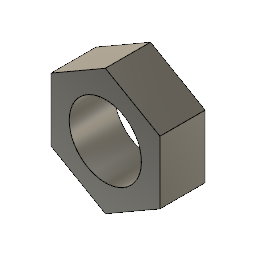
assembly v43 (Autodesk Fusion 360 archive; units mm, degrees)
design "nut"
Autodesk Fusion 360 part; units mm, degrees
sketch "Sketch1" plane through (0, 0, 0) normal (0, 1, 0) x (1, 0, 0)
  circle A0 centre (0, 0) radius 1.75
  line L0 (2.65, 1.53) -> (0, 3.06)
  line L1 (0, 3.06) -> (-2.65, 1.53)
  line L2 (-2.65, 1.53) -> (-2.65, -1.53)
  line L3 (-2.65, -1.53) -> (0, -3.06)
  line L4 (0, -3.06) -> (2.65, -1.53)
  line L5 (2.65, -1.53) -> (2.65, 1.53)
  dimension "d1" = 3.5
  dimension "d2" = 5.3
  constraint coincident A0.centre origin
  measures "d1" diameter of A0
  measures "d2" distance of L2 L5
extrude "Extrude1" add sketch "Sketch1" along normal blind 2.2

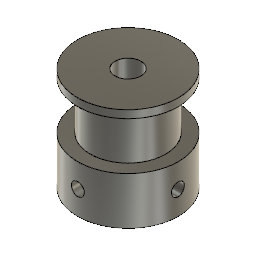
design "motor pulley"
Autodesk Fusion 360 part; units mm, degrees
sketch "Sketch1" plane through (0, 0, 0) normal (0, 0, 1) x (1, 0, 0)
  circle A0 centre (0, 0) radius 7.85
  circle A1 centre (0, 0) radius 2
  dimension "d1" = 15.7
  dimension "d4" = 4
  constraint coincident A0.centre A1.centre
  constraint concentric A0 A1
  measures "d1" diameter of A0
  measures "d4" diameter of A1
extrude "Extrude1" add sketch "Sketch1" along normal blind 16 makes body 1
copy_body "Body->Comp1" bodies 1 removing the originals makes body 2 in component "Component"
sketch "Sketch3" plane through (0, 0, 16) normal (0, 0, 1) x (-1, 0, 0)
  circle A0 centre (0, 0) radius 2
  circle A1 centre (0, 0) radius 7.85
  circle A2 centre (0, 0) radius 5.85
  dimension "d6" = 2
  constraint coincident A0.centre A1.centre
  measures "d6" distance of A1 A2
extrude "Extrude1'" cut sketch "Sketch3" against normal blind 7.4 from surface at -1.2 contours A1 bodies 2 in component "Component"
sketch "Sketch4" plane through (0, 0, 0) normal (0, 1, 0) x (1, 0, 0)
  circle A0 centre (0, -3.7) radius 1
  line L0 (0, 0) -> (0, -7.4) construction
  dimension "d10" = 7.4
  dimension "d18" = 2
  constraint coincident L0.start origin
  constraint vertical L0
  constraint coincident A0.centre L0
  constraint midpoint A0.centre L0
  measures "d10" distance of L0.start L0.end
  measures "d18" diameter of A0
extrude "Extrude3" cut sketch "Sketch4" against normal blind 17 bodies 2 in component "Component"
sketch "Sketch5" plane through (0, 0, 0) normal (1, 0, 0) x (0, 1, 0)
  circle A0 centre (-0.0371, 3.6862) radius 1
  dimension "d15" = 2
  measures "d15" diameter of A0
extrude "Extrude4" cut sketch "Sketch5" along normal blind 14.5 bodies 2 in component "Component"
component "Component" placed x (1, 0, 0) y (0, 1, 0) z (0, 0, 1) at (0, 0, 0)

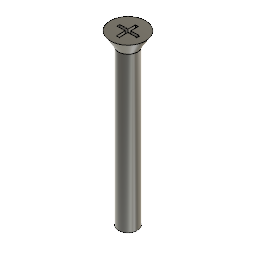
design "screw"
Autodesk Fusion 360 part; units mm, degrees
sketch "Sketch1" plane through (0, 0, 0) normal (0, 0, 1) x (1, 0, 0)
  circle A0 centre (0, 0) radius 1.4
  dimension "d1" = 2.8
  constraint coincident A0.centre origin
  measures "d1" diameter of A0
extrude "Extrude1" add sketch "Sketch1" along normal blind 24.7
sketch "Sketch2" plane through (0, 0, 24.7) normal (0, 0, 1) x (-1, 0, 0)
  circle A0 centre (0, 0) radius 1.4
  circle A1 centre (0, 0) radius 2.6
  dimension "d4" = 5.2
  constraint coincident A0.centre A1.centre
  measures "d4" diameter of A1
extrude "Extrude2" add sketch "Sketch2" against normal blind 2
chamfer "Chamfer1" distance 1.2 distance2 2 1 edges at (2.4241, -0.9402, 22.7) measured on face at (-2.1851, 0.1987, 22.7)
sketch "Sketch3" plane through (0, 0, 24.7) normal (0, 0, 1) x (-1, 0, 0)
  circle A0 centre (0, 0) radius 2.6
  line L0 (-0.2, 1.5) -> (0.2, 1.5)
  line L1 (0.2, 1.5) -> (0.2, -1.3)
  line L2 (0.2, -1.3) -> (-0.2, -1.3)
  line L3 (-0.2, -1.3) -> (-0.2, 1.5)
  line L4 (-1.5, 0.2024) -> (1.4, 0.2024)
  line L5 (1.4, 0.2024) -> (1.4, -0.1976)
  line L6 (1.4, -0.1976) -> (-1.5, -0.1976)
  line L7 (-1.5, -0.1976) -> (-1.5, 0.2024)
  line L8 (-2.6, 0.0024) -> (2.6, 0.0024) construction
  line L9 (0, 2.6) -> (0, -2.6) construction
  dimension "d10" = 0.2
  dimension "d11" = 0.2
  dimension "d12" = 0.2
  dimension "d13" = 0.2
  constraint horizontal L0
  constraint vertical L1
  constraint horizontal L2
  constraint vertical L3
  constraint horizontal L4
  constraint vertical L5
  constraint horizontal L6
  constraint vertical L7
  constraint coincident A0 L8.start
  constraint coincident A0 L8.end
  constraint perpendicular L5 L8
  constraint coincident A0 L9.start
  constraint coincident A0 L9.end
  constraint perpendicular L0 L9
  measures "d10" distance of L5.end L8
  measures "d11" distance of L4.start L8
  measures "d12" distance of L3 L9
  measures "d13" distance of L1.end L9
extrude "Extrude3" cut sketch "Sketch3" against normal blind 1 contours L0 L1 L3 L4 | L1 L3 L4 L6 | L3 L4 L6 L7 | L1 L4 L5 L6 | L1 L2 L3 L6
equation "d10 = d11"
equation "d12 = d11"
equation "d13 = d12"

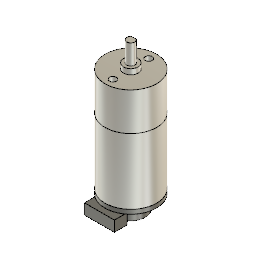
design "motor"
Autodesk Fusion 360 part; units mm, degrees
sketch "Sketch1" plane through (0, 0, 0) normal (0, 0, 1) x (1, 0, 0)
  circle A0 centre (0, 0) radius 12
  dimension "d1" = 24
  constraint coincident A0.centre origin
  measures "d1" diameter of A0
extrude "Extrude1" add sketch "Sketch1" along normal blind 30.5 makes body 1 in component "Component"
sketch "Sketch2" plane through (0, 0, 30.5) normal (0, 0, 1) x (-1, 0, 0)
  circle A0 centre (0, 0) radius 12
  circle A1 centre (0, 0) radius 12.5
  dimension "d4" = 0.5
  constraint concentric A0 A1
  measures "d4" distance of A0 A1
extrude "Extrude1'" add sketch "Sketch2" along normal blind 17.6 separate body contours A0 makes body 2 in component "Component'"
sketch "Sketch3" plane through (0, 0, 48.1) normal (0, 0, 1) x (-1, 0, 0)
  circle A0 centre (0, 0) radius 12
  circle A1 centre (0, 0) radius 3.4
  circle A2 centre (0, 0) radius 1.9
  dimension "d7" = 6.8
  dimension "d8" = 3.8
  constraint coincident A0.centre A1.centre
  measures "d7" diameter of A1
  measures "d8" diameter of A2
extrude "Extrude2" add sketch "Sketch3" along normal blind 2.5 separate body contours A1 makes body 3 in component "Component'"
sketch "Sketch4" plane through (0, 0, 48.1) normal (0, 0, 1) x (-1, 0, 0)
  circle A0 centre (0, 0) radius 12
  circle A1 centre (0, 0) radius 1.9
  circle A2 centre (0, 8.35) radius 1.6
  circle A3 centre (0, -8.35) radius 1.6
  line L0 (0, -8.35) -> (0, 0) construction
  line L1 (0, 0) -> (0, 8.35) construction
  dimension "d13" = 3.8
  dimension "d24" = 3.2
  dimension "d25" = 3.2
  dimension "d27" = 8.35
  dimension "d29" = 8.35
  dimension "d30" = 16
  constraint concentric A0 A1
  constraint coincident A3.centre L0.start
  constraint coincident A0.centre A1.centre
  constraint vertical L0
  constraint parallel L0 L1
  constraint coincident A2.centre L1.end
  measures "d13" diameter of A1
  measures "d24" diameter of A3
  measures "d25" diameter of A2
  measures "d27" distance of A0.centre A3.centre
  measures "d29" distance of A0.centre A2.centre
extrude "Extrude4" add sketch "Sketch4" along normal blind 11.8 contours A1 bodies 2 3 in component "Component'"
sketch "Sketch5" plane through (0, 0, 59.9) normal (0, 0, 1) x (-1, 0, 0)
  circle A0 centre (0, 0) radius 1.9
  line L0 (0, 0) -> (0, 1.9) construction
  line L1 (0, 0) -> (0, -1.9) construction
  circle A1 centre (0, 0) radius 1.9 construction
  line L2 (1.1662, -1.5) -> (-1.1662, -1.5)
  dimension "d16" = 3.4
  constraint coincident A0.centre L0.start
  constraint coincident A0 L0.end
  constraint vertical L0
  constraint coincident A0 L1.end
  constraint parallel L0 L1
  constraint coincident L1.end A1
  constraint coincident A1 L2.start
  constraint coincident A0 L2.end
  constraint perpendicular L1 L2
  measures "d16" distance of L0.end L2
extrude "Extrude5" cut sketch "Sketch5" against normal blind 8 contours A0 L2 picked at (-0.3114, -1.5515) bodies 2 in component "Component'"
sketch "Sketch6" plane through (0, 0, 0) normal (0, 0, -1) x (1, 0, 0)
  circle A0 centre (0, 0) radius 12
  circle A1 centre (0, 0) radius 12
  constraint coincident A0.centre A1.centre
extrude "Extrude1''" add sketch "Sketch6" along normal blind 2 separate body makes body 4 in component "Component''"
sketch "Sketch7" plane through (0, 0, -2) normal (0, 0, -1) x (1, 0, 0)
  circle A0 centre (0, 0) radius 12
  circle A1 centre (0, 0) radius 0.9
  dimension "d21" = 1.8
  constraint coincident A0.centre A1.centre
  measures "d21" diameter of A1
extrude "Extrude2'" add sketch "Sketch7" along normal blind 8 contours A1 bodies 4 in component "Component''"
extrude "Extrude6" cut sketch "Sketch4" against normal blind 10 contours A2 | A3 bodies 2 in component "Component'"
sketch "Sketch8" plane through (0, 0, -10) normal (0, 0, -1) x (1, 0, 0)
  circle A0 centre (0, 0) radius 0.9
  circle A1 centre (0, 0) radius 6.65
  dimension "d33" = 13.3
  constraint coincident A0.centre A1.centre
  measures "d33" diameter of A1
extrude "Extrude3" add sketch "Sketch8" against normal blind 4.5 from surface at -1.5 bodies 4 in component "Component''"
sketch "Sketch9" plane through (0, 0, -2) normal (0, 0, -1) x (1, 0, 0)
  circle A0 centre (0, 0) radius 0.9
  circle A1 centre (0, 0) radius 12
  line L0 (-7, 14.65) -> (7, 14.65)
  line L1 (7, 14.65) -> (7, 8.65)
  line L2 (7, 8.65) -> (-7, 8.65)
  line L3 (-7, 8.65) -> (-7, 14.65)
  line L4 (0, 0) -> (0, 12) construction
  circle A2 centre (0, 0) radius 6.65 construction
  line L5 (-7, 6.65) -> (7.5, 6.65)
  circle A3 centre (0, 0) radius 6.65
  dimension "d37" = 7
  dimension "d38" = 7
  dimension "d39" = 2
  dimension "d40" = 6
  constraint horizontal L0
  constraint vertical L1
  constraint horizontal L2
  constraint vertical L3
  constraint coincident A0.centre A1.centre
  constraint coincident A1 L4.end
  constraint perpendicular L0 L4
  constraint perpendicular L4 L5
  constraint tangent A2 L5
  constraint tangent A2 A3
  measures "d37" distance of L1.end L4
  measures "d38" horizontal distance of L2.end L4.end
  measures "d39" distance of L2 L5
  measures "d40" distance of L0.end L1.end
extrude "Extrude4'" add sketch "Sketch9" along normal blind 5 contours A1 L1 L2 L3 | A1 L0 L1 L3 picked at (0.2766, 9.7571) bodies 4 in component "Component''"
component "Component" placed x (1, 0, 0) y (0, 1, 0) z (0, 0, 1) at (0, 0, 0)
component "Component'" placed x (1, 0, 0) y (0, 1, 0) z (0, 0, 1) at (0, 0, 0)
component "Component''" placed x (1, 0, 0) y (0, 1, 0) z (0, 0, 1) at (0, 0, 0)
equation "d14 = 2.5 mm + 9.3 mm"
equation "d25 = d24"
equation "d29 = d27"
equation "d38 = d37"
